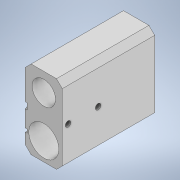
# Autodesk Inventor part: laser holder2
Saved by Autodesk Inventor 2022 (Build 260153000, 153)
## iProperties
Created: 2021-04-14
Part Number: laser holder2
Material: Generic
Document SubType Name: Modeling
Designer: chris
Density: 1 g/cm^3
Appearance: Default
Author: chris
Autodesk Inventor part; units mm, degrees
ref_plane "YZ Plane" through (0, 0, 0) normal (1, 0, 0) x (0, 1, 0)
ref_plane "XZ Plane" through (0, 0, 0) normal (0, 1, 0) x (-1, 0, 0)
ref_plane "XY Plane" through (0, 0, 0) normal (0, 0, 1) x (1, 0, 0)
sketch "Sketch1" plane through (0, 0, 0) normal (0, 0, 1) x (1, 0, 0)
  circle A0 centre (0, 11.43) radius 6.425
  circle A1 centre (0, -11.43) radius 8.25
  line L0 (0, -11.43) -> (0, 11.43)
  line L1 (-10.16, 21.59) -> (-10.16, -21.59)
  line L2 (-10.16, -21.59) -> (10.16, -21.59)
  line L3 (10.16, -21.59) -> (10.16, 21.59)
  line L4 (10.16, 21.59) -> (-10.16, 21.59)
  point P0 (0, 0)
  point P1 (0, 0)
  point P2 (-10.16, 0)
  point P3 (0, -21.59)
  dimension "d0" = 12.85
  dimension "d1" = 16.5
  dimension "d2" = 22.86
  dimension "d3" = 43.18
  dimension "d4" = 20.32
  constraints: 10 end point, 3 midpoint, 3 perpendicular, 2 centre point, 2 vertical, 2 vertical alignment, 1 coincident, 1 horizontal alignment
  measures "d0" diameter of A0
  measures "d1" diameter of A1
  measures "d2" distance of L0.end L0.start
  measures "d3" distance of L1.start L1.end
  measures "d4" distance of L1.end L2.end
extrude "Extrusion1" add sketch "Sketch1" along normal blind 50.8
sketch "Sketch2" plane through (10.16, -21.59, 0) normal (1, 0, 0) x (0, 0, -1)
  line L0 (0, 0) -> (0, 43.18) projected
  line L1 (0, 43.18) -> (-50.8, 43.18) projected
  line L2 (-50.8, 0) -> (-50.8, 43.18) projected
  line L3 (0, 0) -> (-50.8, 0) projected
  circle A0 centre (-47.625, 21.59) radius 1.524
  circle A1 centre (-31.115, 21.59) radius 1.524
  point P0 (0, 21.59)
  point P1 (-50.8, 21.59)
  dimension "d7" = 3.048
  dimension "d8" = 3.048
  dimension "d9" = 16.51
  dimension "d10" = 3.175
  constraints: 2 centre point, 1 horizontal alignment, 1 midpoint
  measures "d7" diameter of A0
  measures "d8" diameter of A1
  measures "d9" distance of A1.centre A0.centre
  measures "d10" distance from line of L2 A0.centre
extrude "Extrusion2" cut sketch "Sketch2" against normal blind 6.35 contours A0 | A1
chamfer "Chamfer1" distance 3.175 angle 45 4 edges at (10.16, 21.59, 25.4) (-10.16, 21.59, 25.4) (10.16, -21.59, 25.4) (-10.16, -21.59, 25.4)
sketch "Sketch3" plane through (-6.985, -21.59, 0) normal (0, -1, 0) x (1, 0, 0)
  line L0 (10.5931, 39.2076) -> (10.5931, 34.27) construction
  line L1 (10.5931, 34.27) -> (-9.3507, 34.27) construction
  line L2 (-9.3507, 34.27) -> (-9.3507, 39.2076) construction
  line L3 (-9.3507, 39.2076) -> (10.5931, 39.2076) construction
  line L4 (0, 0) -> (0, 50.8) projected
  line L5 (0, 0) -> (13.97, 0) projected
  line L6 (13.97, 50.8) -> (13.97, 0) projected
  line L7 (0, 50.8) -> (13.97, 50.8) projected
  line L8 (0, 50.8) -> (0, 0) projected
  line L9 (17.145, 46.101) -> (10.795, 46.101) projected
  line L10 (0, 36.8) -> (13.97, 46.101)
  line L11 (-0.5542, 37.6324) -> (13.4158, 46.9334)
  line L12 (0.5542, 35.9676) -> (14.5242, 45.2686)
  line L13 (15.6348, 47.2094) -> (13.97, 46.101)
  line L14 (17.145, 46.101) -> (10.795, 46.101) projected
  line L15 (14.5242, 45.2686) -> (16.189, 46.377)
  line L16 (16.189, 46.377) -> (15.0806, 48.0418)
  line L17 (15.0806, 48.0418) -> (13.4158, 46.9334)
  line L18 (0, 36.8) -> (-1.6648, 35.6916)
  line L19 (0.5542, 35.9676) -> (-1.1106, 34.8592)
  line L20 (-1.1106, 34.8592) -> (-2.219, 36.524)
  line L21 (-2.219, 36.524) -> (-0.5542, 37.6324)
  line L22 (10.4728, 34.2897) -> (4.3768, 36.31)
  line L23 (4.3768, 36.31) -> (4.3768, 37.1573)
  line L24 (4.3768, 37.1573) -> (10.4728, 39.1776)
  line L25 (10.4728, 39.1776) -> (10.4728, 38.2401)
  line L26 (10.4728, 38.2401) -> (5.595, 36.661)
  line L27 (5.595, 36.661) -> (10.4728, 35.0969)
  line L28 (10.4728, 35.0969) -> (10.4728, 34.2897)
  line L29 (5.5298, 32.5602) -> (4.3768, 32.5602)
  line L30 (4.3768, 32.5602) -> (4.3768, 33.7182)
  line L31 (4.3768, 33.7182) -> (5.5298, 33.7182)
  line L32 (5.5298, 33.7182) -> (5.5298, 32.5602)
  line L33 (4.3768, 30.4045) -> (4.3768, 31.332)
  line L34 (4.3768, 31.332) -> (10.4728, 31.332)
  line L35 (10.4728, 31.332) -> (10.4728, 30.4045)
  line L36 (10.4728, 30.4045) -> (4.3768, 30.4045)
  line L37 (5.5298, 28.0183) -> (4.3768, 28.0183)
  line L38 (4.3768, 28.0183) -> (4.3768, 29.1763)
  line L39 (4.3768, 29.1763) -> (5.5298, 29.1763)
  line L40 (5.5298, 29.1763) -> (5.5298, 28.0183)
  line L41 (5.1839, 22.9349) -> (4.3768, 22.9349)
  line L42 (4.3768, 22.9349) -> (4.3768, 27.2914)
  line L43 (4.3768, 27.2914) -> (5.1238, 27.2914)
  line L44 (5.1238, 27.2914) -> (9.6506, 24.083)
  line L45 (9.6506, 24.083) -> (9.6506, 27.146)
  line L46 (9.6506, 27.146) -> (10.4327, 27.146)
  line L47 (10.4327, 27.146) -> (10.4327, 23.0302)
  line L48 (10.4327, 23.0302) -> (9.8261, 23.0302)
  line L49 (9.8261, 23.0302) -> (5.1839, 26.2737)
  line L50 (5.1839, 26.2737) -> (5.1839, 22.9349)
  line L51 (5.5298, 21.0299) -> (4.3768, 21.0299)
  line L52 (4.3768, 21.0299) -> (4.3768, 22.188)
  line L53 (4.3768, 22.188) -> (5.5298, 22.188)
  line L54 (5.5298, 22.188) -> (5.5298, 21.0299)
  line L55 (4.3768, 18.8743) -> (4.3768, 19.8017)
  line L56 (4.3768, 19.8017) -> (10.4728, 19.8017)
  line L57 (10.4728, 19.8017) -> (10.4728, 18.8743)
  line L58 (10.4728, 18.8743) -> (4.3768, 18.8743)
  line L59 (5.5298, 16.488) -> (4.3768, 16.488)
  line L60 (4.3768, 16.488) -> (4.3768, 17.6461)
  line L61 (4.3768, 17.6461) -> (5.5298, 17.6461)
  line L62 (5.5298, 17.6461) -> (5.5298, 16.488)
  spline S0 degree 2 poles (4.2565, 13.1292) (4.2565, 14.3173) (6.0913, 15.6358) (7.4098, 15.6358) knots 0 0 0 1 2 2 2
  spline S1 degree 2 poles (7.4098, 15.6358) (8.7834, 15.6358) (10.5931, 14.2521) (10.5931, 13.1091) knots 0 0 0 1 2 2 2
  spline S2 degree 2 poles (10.5931, 13.1091) (10.5931, 11.9611) (8.8084, 10.5875) (7.4749, 10.5875) knots 0 0 0 1 2 2 2
  spline S3 degree 2 poles (7.4749, 10.5875) (6.1865, 10.5875) (4.2565, 11.921) (4.2565, 13.1292) knots 0 0 0 1 2 2 2
  spline S4 degree 2 poles (5.0385, 13.1142) (5.0385, 12.3873) (6.3871, 11.5501) (7.4749, 11.5501) knots 0 0 0 1 2 2 2
  spline S5 degree 2 poles (7.4749, 11.5501) (8.5878, 11.5501) (9.806, 12.4123) (9.806, 13.1142) knots 0 0 0 1 2 2 2
  spline S6 degree 2 poles (9.806, 13.1142) (9.806, 13.821) (8.4926, 14.6733) (7.4047, 14.6733) knots 0 0 0 1 2 2 2
  spline S7 degree 2 poles (7.4047, 14.6733) (6.3369, 14.6733) (5.0385, 13.816) (5.0385, 13.1142) knots 0 0 0 1 2 2 2
  line L63 (5.5298, 8.5021) -> (4.3768, 8.5021)
  line L64 (4.3768, 8.5021) -> (4.3768, 9.6601)
  line L65 (4.3768, 9.6601) -> (5.5298, 9.6601)
  line L66 (5.5298, 9.6601) -> (5.5298, 8.5021)
  line L67 (4.3768, 2.7369) -> (4.3768, 3.6092)
  line L68 (4.3768, 3.6092) -> (9.5303, 6.5118)
  line L69 (9.5303, 6.5118) -> (9.2396, 6.5068)
  spline S8 degree 2 poles (9.2396, 6.5068) (8.9889, 6.4918) (8.8586, 6.4918) knots 0 0 0 1 1 1
  line L70 (8.8586, 6.4918) -> (4.3768, 6.4918)
  line L71 (4.3768, 6.4918) -> (4.3768, 7.2738)
  line L72 (4.3768, 7.2738) -> (10.4728, 7.2738)
  line L73 (10.4728, 7.2738) -> (10.4728, 6.201)
  line L74 (10.4728, 6.201) -> (5.6551, 3.4939)
  line L75 (5.6551, 3.4939) -> (5.976, 3.4989)
  spline S9 degree 2 poles (5.976, 3.4989) (6.2166, 3.509) (6.4071, 3.509) knots 0 0 0 1 1 1
  line L76 (6.4071, 3.509) -> (10.4728, 3.509)
  line L77 (10.4728, 3.509) -> (10.4728, 2.7369)
  line L78 (10.4728, 2.7369) -> (4.3768, 2.7369)
  point P0 (6.985, 0)
  point P1 (0, 35.5986)
  point P2 (0, 38.0014)
  point P3 (13.97, 47.3024)
  point P4 (13.97, 44.8996)
  dimension "d18" = 14
  dimension "d19" = 1
  dimension "d20" = 1
  constraints: 22 end point, 4 perpendicular, 3 parallel, 1 midpoint, 1 point on line, 2 other
  measures "d18" distance from line of L7 L10.start
  measures "d19" distance between parallel lines of L10 L11
  measures "d20" distance between parallel lines of L10 L12
extrude "Extrusion3" cut sketch "Sketch3" against normal blind 1 contours L19 L20 L18 L4 | L4 L10 L6 L12 L19 | L18 L20 L21 L11 L4 | L4 L11 L9 L10 | L6 L9 L15 L12 | L9 L11 L17 L6 | L13 L16 L15 L9 | L6 L17 L16 L13 | L22 L23 L24 L25 L26 L27 L28 | L29 L30 L31 L32 | L33 L34 L35 L36 | L37 L38 L39 L40 | L41 L42 L43 L44 L45 L46 L47 L48 L49 L50 | L51 L52 L53 L54 | L55 L56 L57 L58 | L59 L60 L61 L62 | S0 S1 S2 S3 | L63 L64 L65 L66 | L67 L68 L69 S8 L70 L71 L72 L73 L74 L75 S9 L76 L77 L78
extrude "Extrusion4" cut sketch "Sketch3" against normal blind 2 contours L19 L20 L18 L4 | L18 L20 L21 L11 L4 | L6 L9 L15 L12 | L13 L16 L15 L9 | L6 L17 L16 L13
fillet "Fillet1" radius 3.175 2 edges at (6.985, -20.59, 46.101) (-6.985, -20.59, 36.8)
sketch "Sketch4" plane through (-10.16, -18.415, 0) normal (-1, 0, 0) x (0, 0, 1)
  line L0 (50.8, 0) -> (0, 0) projected
  line L1 (50.8, 36.83) -> (50.8, 0) projected
  line L2 (0, 36.83) -> (50.8, 36.83) projected
  line L3 (0, 36.83) -> (0, 0) projected
  circle A0 centre (40.8, 6.985) radius 2
  circle A1 centre (9.5697, 6.985) radius 2
  line L4 (50.8, 23.42) -> (0, 23.42) projected
  line L5 (42.8, 23.42) -> (25.4, 32.305)
  line L6 (0, 36.27) -> (0, 23.42) projected
  line L7 (42.8, 23.42) -> (50.8, 19.3349)
  line L8 (0, 33.305) -> (25.6405, 33.305)
  line L9 (25.6405, 33.305) -> (43.2548, 24.3106)
  line L10 (43.2548, 24.3106) -> (51.2548, 20.2255)
  line L11 (0, 31.23) -> (25.1595, 31.23)
  line L12 (24.4905, 30.5238) -> (41.8905, 21.6388)
  line L13 (41.8905, 21.6388) -> (49.8905, 17.5537)
  line L14 (24.4905, 30.5238) -> (21.0022, 32.305)
  line L15 (49.8905, 17.5537) -> (59.7926, 12.4974)
  line L16 (59.7926, 6.985) -> (-8.4324, 6.985)
  line L17 (59.7926, 5.985) -> (-8.4324, 5.985)
  line L18 (59.7926, 7.985) -> (-8.4324, 7.985)
  line L19 (33.1905, 12.4224) -> (7.5697, 17.4787)
  circle A2 centre (31.115, 18.415) radius 1.524 projected
  line L20 (33.1905, 22.5351) -> (7.5697, 17.4787)
  line L21 (33.1905, 22.5351) -> (19.9436, 17.4787)
  line L22 (33.1905, 12.4224) -> (19.9436, 17.4787)
  point P0 (0, 18.415)
  point P1 (0, 33.305)
  point P2 (23.1074, 31.23)
  point P3 (50.8, 17.0893)
  point P4 (50.8, 20.4578)
  point P5 (50.8, 5.985)
  point P6 (50.8, 7.985)
  point P7 (0, 7.985)
  point P8 (0, 5.985)
  dimension "d26" = 4
  dimension "d27" = 10
  dimension "d28" = 4
  dimension "d33" = 1
  dimension "d35" = 2
  dimension "d36" = 1
  dimension "d37" = 2
  constraints: 34 end point, 3 parallel, 2 centre point, 2 point on line, 1 horizontal, 2 other
  measures "d26" diameter of A0
  measures "d27" distance from line of L1 A0.centre
  measures "d28" diameter of A1
  measures "d33" distance between parallel lines of L5 L9
  measures "d35" distance between parallel lines of L5 L12
  measures "d36" distance between parallel lines of L16 L17
  measures "d37" distance between parallel lines of L17 L18
extrude "Extrusion5" cut sketch "Sketch4" against normal blind 1 contours L17 A0 L16 L1 | L3 L16 A1 L17 | L16 A0 L18 L1 | L17 A0 L16 | L3 L18 A1 L16 | A1 L16 L17 | L16 A0 L18 | L17 A1 L16 A0 | A1 L18 L16 | L15 L13 L12 L4 L7 L1 | L16 A1 L18 A0 | L7 L4 L10 L1 | L3 L8 L9 L10 L4 L12 L14 L11 | L19 L20 L21 L22
body "Solid1"
